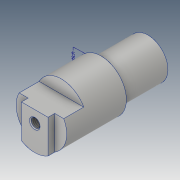
# Autodesk Inventor part: 200-20-ROCKER-CONNECTOR-01
Saved by Autodesk Inventor 2018.2 (Build 222227000, 227)
## iProperties
Manager: feesmrt
Company: FRANC0R
Created: 2017-10-30
Part Number: 200-20-ROCKER-CONNECTOR-01
Material: Aluminium 6061
Document SubType Name: Modeling
Designer: feesmrt
Density: 2.7 g/cm^3
Appearance: Aluminium - flach
Project: Rescue Robot
Cost Center: -
Description: Rocker Profile Connector
Engineer: feesmrt
Authority: feesmrt
Stock Number: 200-20-ROCKER-CONNECTOR-01
Mass: 197.92 g
Surface Area: 134.643 cm^2
Volume: 73.3037 cm^3
Author: feesmrt
Title: Rocker Profile Connector
Subject: Rescue Robot
Revision Number: 1
Autodesk Inventor part; units mm, degrees
ref_plane "YZ Plane" through (0, 0, 0) normal (1, 0, 0) x (0, 1, 0)
ref_plane "XZ Plane" through (0, 0, 0) normal (0, 1, 0) x (-1, 0, 0)
ref_plane "XY Plane" through (0, 0, 0) normal (0, 0, 1) x (1, 0, 0)
derived "200-10-ROCKER-BEARING-01.ipt"
sketch "Skizze_Lagersitz" plane through (0, 0, 0) normal (1, 0, 0) x (0, 1, 0)
  line L0 (-12.5, 36) -> (17.5, 36)
  line L1 (-12.5, -36) -> (-12.5, 36)
  line L2 (-17.5, 31) -> (-12.5, 31)
  line L3 (-17.5, -31) -> (-17.5, 31)
  line L4 (-32.5, 22.5) -> (-17.5, 22.5)
  line L5 (-32.5, -22.5) -> (-17.5, -22.5)
  line L6 (-17.5, -31) -> (-12.5, -31)
  line L7 (-12.5, -36) -> (17.5, -36)
  line L8 (32.5, 50) -> (32.5, -50)
  line L9 (30, -50) -> (30, 0)
  line L10 (-32.5, -22.5) -> (-32.5, 22.5)
  line L11 (-32.5, 50) -> (-32.5, -50)
  line L12 (-32.5, -50) -> (-32.5, 50)
  line L13 (-12.5, -36) -> (-12.5, 36)
  line L14 (17.5, -37.5) -> (17.5, 37.5)
  line L15 (17.5, 37.5) -> (32.5, 37.5)
  point P0 (0, 0)
  point P1 (30, 86)
  point P2 (30, 14)
  point P3 (-30, 32)
  point P4 (-30, 68)
  point P5 (32.5, 36)
  point P6 (32.5, -36)
sketch "Skizze4" plane through (0, 0, 0) normal (1, 0, 0) x (0, 1, 0)
  line L0 (-81.26, 0) -> (51.46, 0) projected
  line L1 (-12.5, -36) -> (-12.5, 36) construction
  line L2 (-32.5, -22.5) -> (-32.5, 22.5) construction
  line L3 (22.7, 0) -> (22.7, 15)
  line L4 (22.7, 15) -> (-12.5, 15)
  line L5 (17.7, 0) -> (17.7, 36) construction
  line L6 (-12.5, 15) -> (-12.5, 19)
  line L7 (-12.5, 19) -> (-62.3, 19)
  line L8 (-62.3, 0) -> (22.7, 0)
  line L9 (-62.3, 19) -> (-62.3, 0)
  line L10 (-12.5, 36) -> (17.5, 36) construction
  point P0 (0, 0)
  dimension "d3" = 30.2
  dimension "d4" = 5
  dimension "d5" = 30
  dimension "d6" = 38
  dimension "d7" = 85
  constraints: 14 end point, 6 point on line, 2 horizontal, 2 vertical, 1 collinear, 1 perpendicular
  measures "d3" distance between parallel lines of L5 L1
  measures "d4" distance between parallel lines of L3 L5
  measures "d5" diameter of L4 L0
  measures "d6" diameter of L7 L0
  measures "d7" distance from line of L7.end L3
revolve "Grundkoerper" add sketch "Skizze4" angle 360 about axis through (0, 0, 0) along (0, 1, 0)
sketch "Skizze11" plane through (0, -62.3, 0) normal (0, -1, 0) x (1, 0, 0)
  circle A0 centre (0, 0) radius 19 projected
hole "M6x12_CubeConn" at (0, -62.3, 0) direction (0, 1, 0) diameter 6.647 depth 25 tip angle 118 countersink diameter 8 countersink angle 90 thread size "M8x1.25" class "6H" standard "ISO Metric profile"
sketch "Skizze14" plane through (0, 22.7, 0) normal (0, 1, 0) x (1, 0, 0)
  circle A0 centre (0, 0) radius 15 construction
  constraints: 1 coincident
hole "M6x12_BearingFix" at (0, 22.7, 0) direction (0, -1, 0) diameter 4.917 depth 17.1 tip angle 118 countersink diameter 6 countersink angle 90 thread size "M6x1" class "6H" standard "ISO Metric profile"
sketch "Skizze17" plane through (0, -62.3, 0) normal (0, -1, 0) x (1, 0, 0)
  circle A0 centre (0, 0) radius 19 projected
  line L0 (-26.6, 0) -> (26.6, 0) construction
  line L1 (0, 113.2) -> (0, -77.2) construction
  arc A1 (17.2337, 8) -> (-17.2337, 8) centre (0, 0) ccw projected
  arc A2 (-15.4919, -11) -> (15.4919, -11) centre (0, 0) ccw projected
  line L2 (-10, 16.1555) -> (-10, -16.1555)
  line L3 (10, 16.1555) -> (10, -16.1555)
  dimension "d120" = 20
  constraints: 4 end point, 2 vertical, 6 other
  measures "d120" distance between parallel lines of L2 L3
extrude "Absatz_Torsionssicherung" cut sketch "Skizze17" against normal blind 5 contours A0 L3 | L2 A0
sketch "Skizze18" plane through (0, 0, 0) normal (1, 0, 0) x (0, 1, 0)
  line L0 (-62.3, 19) -> (-12.5, 19) projected
  line L1 (-62.3, -16.1555) -> (-62.3, 16.1555) projected
  line L2 (-62.3, 9) -> (-42.3, 9)
  line L3 (-42.3, 9) -> (-42.3, 19)
  line L4 (-62.3, 16.1555) -> (-62.3, 19) projected
  point P0 (0, 0)
  dimension "d123" = 20
  dimension "d124" = 10
  constraints: 4 end point, 2 point on line, 1 horizontal, 1 perpendicular
  measures "d123" distance between parallel lines of L4 L3
  measures "d124" distance between parallel lines of L0 L2
extrude "Absatz_Differential" cut sketch "Skizze18" along normal through all both and the other way through all
